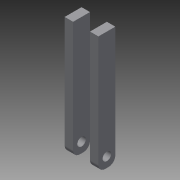
# Autodesk Inventor part: manipulator first link
Saved by Autodesk Inventor 2015 (Build 190159000, 159)
## iProperties
Created: 2014-10-18
Part Number: manipulator first link
Material: Generic
Document SubType Name: Modeling
Designer: ericd_000
Density: 1 g/cm^3
Appearance: Default
Author: ericd_000
Autodesk Inventor part; units mm, degrees
ref_plane "YZ Plane" through (0, 0, 0) normal (1, 0, 0) x (0, 1, 0)
ref_plane "XZ Plane" through (0, 0, 0) normal (0, 1, 0) x (-1, 0, 0)
ref_plane "XY Plane" through (0, 0, 0) normal (0, 0, 1) x (1, 0, 0)
sketch "Sketch1" plane through (0, 0, 0) normal (0, 0, 1) x (1, 0, 0)
  line L0 (-5, 0) -> (5, 0) construction
  line L1 (-5, -5) -> (-10, -5)
  line L2 (-10, -5) -> (-10, 5)
  line L3 (-10, 5) -> (-5, 5)
  line L4 (-5, 5) -> (-5, -5)
  line L5 (10, -5) -> (5, -5)
  line L6 (5, -5) -> (5, 5)
  line L7 (5, 5) -> (10, 5)
  line L8 (10, 5) -> (10, -5)
  point P0 (0, 0)
  point P1 (0, 0)
  dimension "d0" = 10
  dimension "d1" = 5
  dimension "d2" = 5
  dimension "d3" = 10
  dimension "d4" = 10
  constraints: 18 end point, 5 coincident, 4 parallel, 3 horizontal, 3 midpoint, 2 perpendicular
  measures "d0" distance of L0.start L0.end
  measures "d1" distance of L2.end L3.end
  measures "d2" distance of L6.end L7.end
  measures "d3" distance of L1.end L2.end
  measures "d4" distance of L7.end L5.start
extrude "Extrusion1" add sketch "Sketch1" along normal blind 70
fillet "Fillet1" radius 4 4 edges at (7.5, -5, 0) (7.5, 5, 0) (-7.5, -5, 0) (-7.5, 5, 0)
sketch "Sketch2" plane through (10, -5, 70) normal (1, 0, 0) x (0, 0, -1)
  circle A0 centre (64, 5) radius 2.5
  point P0 (70, 5)
  dimension "d8" = 5
  dimension "d9" = 6
  constraints: 1 centre point
  measures "d8" diameter of A0
  measures "d9" distance of A0.centre point (70, 5)
extrude "Extrusion2" cut sketch "Sketch2" against normal up to surface (20 mm away)
body "Solid1"
